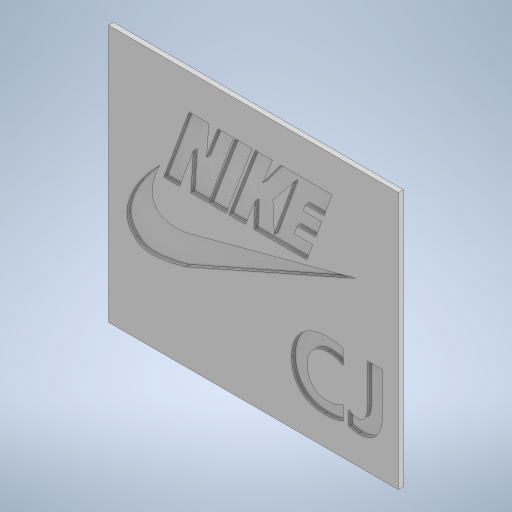
# Autodesk Inventor part: Silueta_nike_nombres
Saved by Autodesk Inventor 2024.2 (Build 282272000, 272)
## iProperties
Created: 2024-03-17
Part Number: Silueta_nike_nombres
Material: Genérico
Document SubType Name: Modeling
Designer: USUARIO
Density: 1 g/cm^3
Appearance: Valor por defecto
Author: USUARIO
Autodesk Inventor part; units mm, degrees
ref_plane "YZ Plane" through (0, 0, 0) normal (1, 0, 0) x (0, 1, 0)
ref_plane "XZ Plane" through (0, 0, 0) normal (0, 1, 0) x (-1, 0, 0)
ref_plane "XY Plane" through (0, 0, 0) normal (0, 0, 1) x (1, 0, 0)
sketch "Boceto1" plane through (0, 0, 0) normal (0, 0, 1) x (1, 0, 0)
  line L0 (-250, -250) -> (250, -250)
  line L1 (250, -250) -> (250, 250)
  line L2 (250, 250) -> (-250, 250)
  line L3 (-250, 250) -> (-250, -250)
  line L4 (-250, -250) -> (250, 250) construction
  line L5 (250, -250) -> (-250, 250) construction
  point P0 (0, 0)
  dimension "d0" = 500
  dimension "d1" = 500
  constraints: 12 end point, 2 midpoint, 2 parallel, 1 horizontal, 1 perpendicular
  measures "d0" distance of L2.end L1.end
  measures "d1" distance of L0.end L1.end
extrude "Extrusión1" add sketch "Boceto1" along normal blind 6
sketch "Boceto4" plane through (0, 0, 6) normal (0, 0, 1) x (1, 0, 0)
  line L0 (-122.9682, 69.533) -> (177.0318, 69.533) construction
  line L1 (177.0318, 69.533) -> (177.0318, -53.8632) construction
  line L2 (177.0318, -53.8632) -> (-122.9682, -53.8632) construction
  line L3 (-122.9682, -53.8632) -> (-122.9682, 69.533) construction
  line L4 (163.4789, 57.5416) -> (-40.9722, 2.948)
  spline S0 degree 4 poles (-40.9722, 2.948) (-59.3478, 1.0194) (-98.1126, -3.325) (-80.4924, 43.1707) (-72.4826, 57.5416) knots 0 0 0 0 0 1 1 1 1 1
  spline S1 degree 4 poles (-72.4826, 57.5416) (-101.0846, 27.8162) (-107.584, 11.7419) (-123.1576, -16.2785) (-102.1609, -32.5927) knots 0 0 0 0 0 1 1 1 1 1
  spline S2 degree 3 poles (-102.1609, -32.5927) (-92.0174, -46.5521) (-57.6708, -37.567) (-40.9722, -32.5927) knots 0 0 0 0 1 1 1 1
  line L5 (-40.9722, -32.5927) -> (163.4789, 57.5416)
  point P0 (0, 0)
  point P1 (-62.9545, 2.949)
  point P2 (-77.976, 12.1095)
  point P3 (-80.9081, 33.7265)
  point P4 (-98.8634, 24.932)
  point P5 (-109.4889, 2.9481)
  point P6 (-111.753, -15.9522)
  point P7 (-88.6041, -39.5543)
  point P8 (-62.956, -38.0886)
  dimension "d19" = 300
  constraints: 4 end point, 16 other
  measures "d19" distance of L1.end L2.end
extrude "Extrusión4" cut sketch "Boceto4" against normal blind 4.5
sketch "Boceto6" plane through (0, 0, 6) normal (0, 0, 1) x (1, 0, 0)
  line L0 (82.2007, -20.2301) -> (276.8192, -20.2301) construction
  line L1 (276.8192, -20.2301) -> (276.8192, -107.8084) construction
  line L2 (276.8192, -107.8084) -> (82.2007, -107.8084) construction
  line L3 (82.2007, -107.8084) -> (82.2007, -20.2301) construction
  spline S0 degree 2 poles (148.6942, -98.7459) (139.9372, -102.9759) (125.8371, -102.9759) knots 0 0 0 1 1 1
  spline S1 degree 2 poles (125.8371, -102.9759) (107.4326, -102.9759) (86.3565, -81.3061) (86.3565, -63.2728) knots 0 0 0 1 2 2 2
  spline S2 degree 2 poles (86.3565, -63.2728) (86.3565, -44.052) (110.03, -20.2301) (128.9539, -20.2301) knots 0 0 0 1 2 2 2
  spline S3 degree 2 poles (128.9539, -20.2301) (140.6794, -20.2301) (148.6942, -23.1243) knots 0 0 0 1 1 1
  line L4 (148.6942, -23.1243) -> (148.6942, -40.4898)
  spline S4 degree 2 poles (148.6942, -40.4898) (140.6794, -35.7403) (130.4382, -35.7403) knots 0 0 0 1 1 1
  spline S5 degree 2 poles (130.4382, -35.7403) (119.158, -35.7403) (105.2805, -49.9147) (105.2805, -62.0112) knots 0 0 0 1 2 2 2
  spline S6 degree 2 poles (105.2805, -62.0112) (105.2805, -73.5882) (118.3417, -87.3915) (129.3992, -87.3915) knots 0 0 0 1 2 2 2
  spline S7 degree 2 poles (129.3992, -87.3915) (139.9372, -87.3915) (148.6942, -82.2709) knots 0 0 0 1 1 1
  line L5 (148.6942, -82.2709) -> (148.6942, -98.7459)
  spline S8 degree 2 poles (196.0411, -69.8034) (196.0411, -85.9073) (181.1246, -102.9759) (167.0244, -102.9759) knots 0 0 0 1 2 2 2
  spline S9 degree 2 poles (167.0244, -102.9759) (160.7165, -102.9759) (155.3732, -100.7496) knots 0 0 0 1 1 1
  line L6 (155.3732, -100.7496) -> (155.3732, -83.9036)
  spline S10 degree 2 poles (155.3732, -83.9036) (159.9744, -87.3915) (165.7629, -87.3915) knots 0 0 0 1 1 1
  spline S11 degree 2 poles (165.7629, -87.3915) (178.082, -87.3915) (178.082, -69.0613) knots 0 0 0 1 1 1
  line L7 (178.082, -69.0613) -> (178.082, -21.5659)
  line L8 (178.082, -21.5659) -> (196.0411, -21.5659)
  line L9 (196.0411, -21.5659) -> (196.0411, -69.8034)
  point P0 (0, 0)
  constraints: 2 other
extrude "Extrusión5" cut sketch "Boceto6" against normal blind 4.5
sketch "Boceto7" plane through (0, 0, 6) normal (0, 0, 1) x (1, 0, 0)
  line L0 (-96.8701, 190.9254) -> (156.7066, 190.9254) construction
  line L1 (156.7066, 190.9254) -> (156.7066, -16.508) construction
  line L2 (156.7066, -16.508) -> (-96.8701, -16.508) construction
  line L3 (-96.8701, -16.508) -> (-96.8701, 190.9254) construction
  line L4 (-67.4617, 47.7989) -> (-48.6104, 47.7989)
  line L5 (-48.6104, 47.7989) -> (-31.9884, 92.9574)
  line L6 (-31.9884, 92.9574) -> (-34.8888, 47.7989)
  line L7 (-34.8888, 47.7989) -> (-13.9857, 47.7989)
  line L8 (-13.9857, 47.7989) -> (16.5477, 130.7517)
  line L9 (16.5477, 130.7517) -> (-2.1497, 130.7517)
  line L10 (-13.3744, 130.7517) -> (-36.9283, 130.7517)
  line L11 (-36.9283, 130.7517) -> (-67.4617, 47.7989)
  line L12 (7.7072, 47.7989) -> (-12.5423, 47.7989)
  line L13 (-12.5423, 47.7989) -> (18.6965, 130.7517)
  line L14 (18.6965, 130.7517) -> (38.946, 130.7517)
  line L15 (38.946, 130.7517) -> (7.7072, 47.7989)
  line L16 (-13.3744, 130.7517) -> (-16.165, 94.0996)
  line L17 (-2.1497, 130.7517) -> (-16.165, 94.0996)
  line L18 (42.7507, 130.7517) -> (63.3753, 130.7517)
  line L19 (63.3753, 130.7517) -> (51.8446, 101.3389)
  line L20 (51.8446, 101.3389) -> (73.7311, 130.7517)
  line L21 (73.7311, 130.7517) -> (135.5179, 130.7517)
  line L22 (135.5179, 130.7517) -> (125.7617, 104.2462)
  line L23 (125.7617, 104.2462) -> (103.1886, 104.2462)
  line L24 (103.1886, 104.2462) -> (100.257, 96.2815)
  line L25 (100.257, 96.2815) -> (122.8301, 96.2815)
  line L26 (122.8301, 96.2815) -> (115.7727, 77.108)
  line L27 (115.7727, 77.108) -> (93.1995, 77.108)
  line L28 (93.1995, 77.108) -> (89.4446, 66.9066)
  line L29 (89.4446, 66.9066) -> (112.0177, 66.9066)
  line L30 (112.0177, 66.9066) -> (104.9845, 47.7989)
  line L31 (104.9845, 47.7989) -> (41.2278, 47.7989)
  line L32 (41.2278, 47.7989) -> (42.6118, 77.7874)
  line L33 (42.6118, 77.7874) -> (30.8554, 47.7989)
  line L34 (11.0305, 47.7989) -> (42.7507, 130.7517)
  line L35 (30.8554, 47.7989) -> (11.0305, 47.7989)
  line L36 (89.4446, 121.013) -> (65.5232, 54.1821)
  line L37 (65.5232, 54.1821) -> (63.9179, 89.2753)
  line L38 (63.9179, 89.2753) -> (89.4446, 121.013)
  point P0 (0, 0)
  constraints: 70 end point, 20 point on line, 10 parallel, 3 horizontal, 2 other
extrude "Extrusión6" cut sketch "Boceto7" against normal blind 4.5
sketch "Boceto8" plane through (0, 0, 6) normal (0, 0, 1) x (1, 0, 0)
  line L0 (-134.2632, 172.8911) -> (215.2572, 172.8911)
  line L1 (215.2572, 172.8911) -> (215.2572, -137.3783)
  line L2 (215.2572, -137.3783) -> (-134.2632, -137.3783)
  line L3 (-134.2632, -137.3783) -> (-134.2632, 172.8911)
  line L4 (250, 250) -> (-250, 250) projected
  line L5 (250, -250) -> (250, 250) projected
  line L6 (-250, 250) -> (250, 250)
  line L7 (250, 250) -> (250, -250)
  line L8 (250, -250) -> (-250, -250)
  line L9 (-250, -250) -> (-250, 250)
  point P0 (0, 0)
  constraints: 16 end point, 4 parallel, 2 horizontal, 2 perpendicular
extrude "Extrusión7" cut sketch "Boceto8" against normal blind 133.25
equation "\"d1\" = d0"
